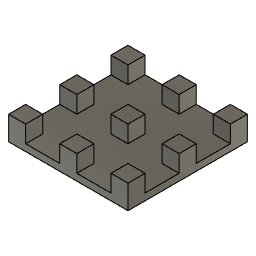
BasePlateTest (Autodesk Fusion 360 design; units mm, degrees)
Autodesk Fusion 360 part; units mm, degrees
sketch "Sketch1" plane through (0, 0, 0) normal (0, 0, 1) x (1, 0, 0)
  line L0 (0, 0) -> (-50, 0)
  line L1 (-50, 0) -> (-50, 50)
  line L2 (-50, 50) -> (0, 50)
  line L3 (0, 50) -> (0, 0)
  line L4 (-45, 45) -> (-47.5, 45)
  line L5 (-47.5, 45) -> (-47.5, 47.5)
  line L6 (-47.5, 47.5) -> (-45, 47.5)
  line L7 (-45, 47.5) -> (-45, 45)
  line L8 (-45, 45) -> (-42.5, 45)
  line L9 (-42.5, 45) -> (-42.5, 42.5)
  line L10 (-42.5, 42.5) -> (-45, 42.5)
  line L11 (-45, 42.5) -> (-45, 45)
  line L12 (-42.5, 42.5) -> (-47.5, 42.5)
  line L13 (-47.5, 42.5) -> (-47.5, 47.5)
  line L14 (-47.5, 47.5) -> (-42.5, 47.5)
  line L15 (-42.5, 47.5) -> (-42.5, 42.5)
  line L16 (-30, 45) -> (-32.5, 45)
  line L17 (-32.5, 45) -> (-32.5, 47.5)
  line L18 (-32.5, 47.5) -> (-30, 47.5)
  line L19 (-30, 47.5) -> (-30, 45)
  line L20 (-32.5, 47.5) -> (-27.5, 47.5)
  line L21 (-27.5, 47.5) -> (-27.5, 42.5)
  line L22 (-27.5, 42.5) -> (-32.5, 42.5)
  line L23 (-32.5, 42.5) -> (-32.5, 47.5)
  line L24 (-15, 45) -> (-17.5, 45)
  line L25 (-17.5, 45) -> (-17.5, 47.5)
  line L26 (-17.5, 47.5) -> (-15, 47.5)
  line L27 (-15, 47.5) -> (-15, 45)
  line L28 (-17.5, 47.5) -> (-12.5, 47.5)
  line L29 (-12.5, 47.5) -> (-12.5, 42.5)
  line L30 (-12.5, 42.5) -> (-17.5, 42.5)
  line L31 (-17.5, 42.5) -> (-17.5, 47.5)
  line L32 (-15, 30) -> (-17.5, 30)
  line L33 (-17.5, 30) -> (-17.5, 32.5)
  line L34 (-17.5, 32.5) -> (-15, 32.5)
  line L35 (-15, 32.5) -> (-15, 30)
  line L36 (-17.5, 32.5) -> (-12.5, 32.5)
  line L37 (-12.5, 32.5) -> (-12.5, 27.5)
  line L38 (-12.5, 27.5) -> (-17.5, 27.5)
  line L39 (-17.5, 27.5) -> (-17.5, 32.5)
  line L40 (-45, 30) -> (-47.5, 30)
  line L41 (-47.5, 30) -> (-47.5, 32.5)
  line L42 (-47.5, 32.5) -> (-45, 32.5)
  line L43 (-45, 32.5) -> (-45, 30)
  line L44 (-47.5, 32.5) -> (-42.5, 32.5)
  line L45 (-42.5, 32.5) -> (-42.5, 27.5)
  line L46 (-42.5, 27.5) -> (-47.5, 27.5)
  line L47 (-47.5, 27.5) -> (-47.5, 32.5)
  line L48 (-30, 30) -> (-32.5, 30)
  line L49 (-32.5, 30) -> (-32.5, 32.5)
  line L50 (-32.5, 32.5) -> (-30, 32.5)
  line L51 (-30, 32.5) -> (-30, 30)
  line L52 (-32.5, 32.5) -> (-27.5, 32.5)
  line L53 (-27.5, 32.5) -> (-27.5, 27.5)
  line L54 (-27.5, 27.5) -> (-32.5, 27.5)
  line L55 (-32.5, 27.5) -> (-32.5, 32.5)
  line L56 (-45, 15) -> (-47.5, 15)
  line L57 (-47.5, 15) -> (-47.5, 17.5)
  line L58 (-47.5, 17.5) -> (-45, 17.5)
  line L59 (-45, 17.5) -> (-45, 15)
  line L60 (-47.5, 17.5) -> (-42.5, 17.5)
  line L61 (-42.5, 17.5) -> (-42.5, 12.5)
  line L62 (-42.5, 12.5) -> (-47.5, 12.5)
  line L63 (-47.5, 12.5) -> (-47.5, 17.5)
  line L64 (-30, 15) -> (-32.5, 15)
  line L65 (-32.5, 15) -> (-32.5, 17.5)
  line L66 (-32.5, 17.5) -> (-30, 17.5)
  line L67 (-30, 17.5) -> (-30, 15)
  line L68 (-32.5, 17.5) -> (-27.5, 17.5)
  line L69 (-27.5, 17.5) -> (-27.5, 12.5)
  line L70 (-27.5, 12.5) -> (-32.5, 12.5)
  line L71 (-32.5, 12.5) -> (-32.5, 17.5)
  line L72 (-15, 15) -> (-17.5, 15)
  line L73 (-17.5, 15) -> (-17.5, 17.5)
  line L74 (-17.5, 17.5) -> (-15, 17.5)
  line L75 (-15, 17.5) -> (-15, 15)
  line L76 (-17.5, 17.5) -> (-12.5, 17.5)
  line L77 (-12.5, 17.5) -> (-12.5, 12.5)
  line L78 (-12.5, 12.5) -> (-17.5, 12.5)
  line L79 (-17.5, 12.5) -> (-17.5, 17.5)
  point P0 (-45, 45)
  point P1 (-30, 45)
  point P2 (-15, 45)
  point P3 (-45, 30)
  point P4 (-30, 30)
  point P5 (-15, 30)
  point P6 (-15, 15)
  point P7 (-30, 15)
  point P8 (-45, 15)
  dimension "d1" = 2.5
  dimension "d2" = 2.5
  dimension "d3" = 2.5
  dimension "d4" = 5
  dimension "d5" = 5
  dimension "d6" = 2.5
  dimension "d7" = 2.5
  dimension "d8" = 5
  dimension "d9" = 5
  dimension "d10" = 2.5
  dimension "d11" = 2.5
  dimension "d12" = 5
  dimension "d13" = 5
  dimension "d14" = 2.5
  dimension "d15" = 2.5
  dimension "d16" = 5
  dimension "d17" = 5
  dimension "d18" = 2.5
  dimension "d19" = 2.5
  dimension "d20" = 5
  dimension "d21" = 5
  constraint horizontal L0
  constraint vertical L1
  constraint horizontal L2
  constraint vertical L3
  constraint coincident L0.start L3.end
  constraint horizontal L4
  constraint vertical L5
  constraint horizontal L6
  constraint vertical L7
  constraint coincident P0 L4.start
  constraint horizontal L8
  constraint vertical L9
  constraint horizontal L10
  constraint vertical L11
  constraint horizontal L12
  constraint vertical L13
  constraint horizontal L14
  constraint vertical L15
  constraint horizontal L16
  constraint vertical L17
  constraint horizontal L18
  constraint vertical L19
  constraint coincident P1 L16.start
  constraint horizontal L20
  constraint vertical L21
  constraint horizontal L22
  constraint vertical L23
  constraint horizontal L24
  constraint vertical L25
  constraint horizontal L26
  constraint vertical L27
  constraint coincident P2 L24.start
  constraint horizontal L28
  constraint vertical L29
  constraint horizontal L30
  constraint vertical L31
  constraint horizontal L32
  constraint vertical L33
  constraint horizontal L34
  constraint vertical L35
  constraint coincident P5 L32.start
  constraint horizontal L36
  constraint vertical L37
  constraint horizontal L38
  constraint vertical L39
  constraint horizontal L40
  constraint vertical L41
  constraint horizontal L42
  constraint vertical L43
  constraint coincident P3 L40.start
  constraint horizontal L44
  constraint vertical L45
  constraint horizontal L46
  constraint vertical L47
  constraint horizontal L48
  constraint vertical L49
  constraint horizontal L50
  constraint vertical L51
  constraint coincident P4 L48.start
  constraint horizontal L52
  constraint vertical L53
  constraint horizontal L54
  constraint vertical L55
  constraint horizontal L56
  constraint vertical L57
  constraint horizontal L58
  constraint vertical L59
  constraint coincident P8 L56.start
  constraint horizontal L60
  constraint vertical L61
  constraint horizontal L62
  constraint vertical L63
  constraint horizontal L64
  constraint vertical L65
  constraint horizontal L66
  constraint vertical L67
  constraint coincident P7 L64.start
  constraint horizontal L68
  constraint vertical L69
  constraint horizontal L70
  constraint vertical L71
  constraint horizontal L72
  constraint vertical L73
  constraint horizontal L74
  constraint vertical L75
  constraint coincident P6 L72.start
  constraint horizontal L76
  constraint vertical L77
  constraint horizontal L78
  constraint vertical L79
  measures "d1" distance of P0 L4.end
  measures "d2" distance of P0 L6.end
  measures "d3" distance of P3 L40.end
  measures "d4" distance of L41.end L44.end
  measures "d5" distance of L41.end L46.end
  measures "d6" distance of P4 L48.end
  measures "d7" distance of P4 L50.end
  measures "d8" distance of L49.end L52.end
  measures "d9" distance of L49.end L54.end
  measures "d10" distance of P8 L56.end
  measures "d11" distance of P8 L58.end
  measures "d12" distance of L57.end L60.end
  measures "d13" distance of L57.end L62.end
  measures "d14" distance of P7 L64.end
  measures "d15" distance of P7 L66.end
  measures "d16" distance of L65.end L68.end
  measures "d17" distance of L65.end L70.end
  measures "d18" distance of P6 L72.end
  measures "d19" distance of P6 L74.end
  measures "d20" distance of L73.end L76.end
  measures "d21" distance of L73.end L78.end
extrude "Extrude1" add sketch "Sketch1" along normal blind 2
extrude "Extrude2" add sketch "Sketch1" along normal blind 7 contours L4 L11 L12 L13 | L4 L5 L6 L7 L13 L14 | L7 L8 L14 L15 | L8 L9 L10 L11 L12 L15 | L16 L19 L20 L21 L22 L23 | L16 L17 L18 L19 L20 L23 | L24 L27 L28 L29 L30 L31 | L24 L25 L26 L27 L28 L31 | L32 L35 L36 L37 L38 L39 | L32 L33 L34 L35 L36 L39 | L40 L43 L44 L45 L46 L47 | L40 L41 L42 L43 L44 L47 | L48 L51 L52 L53 L54 L55 | L48 L49 L50 L51 L52 L55 | L56 L59 L60 L61 L62 L63 | L56 L57 L58 L59 L60 L63 | L64 L67 L68 L69 L70 L71 | L64 L65 L66 L67 L68 L71 | L72 L75 L76 L77 L78 L79 | L72 L73 L74 L75 L76 L79
extrude "Extrude3" add 1 faces at (-50, 16.6667, 0.6667) along direction (-1, 0, 0) blind 5
extrude "Extrude4" cut 1 faces at (-18.3333, 0, 0.6667) along direction (0, 1, 0) blind 12.5
extrude "Extrude5" cut 1 faces at (-55, 25, 1.3333) along direction (1, 0, 0) blind 7.5
extrude "Extrude6" cut 1 faces at (-15.8333, 50, 0.6667) along direction (0, -1, 0) blind 2.5
extrude "Extrude7" cut 1 faces at (0, 35.8333, 0.6667) along direction (-1, 0, 0) blind 12.5
